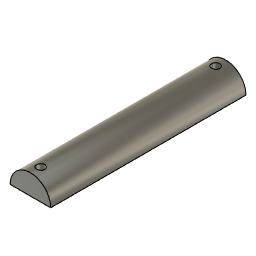
Shaker Fixture v1 (Autodesk Fusion 360 design; units mm, degrees)
Autodesk Fusion 360 part; units mm, degrees
sketch "Sketch1" plane through (0, 0, 0) normal (0, 1, 0) x (1, 0, 0)
  line L0 (0, 0) -> (10, 0)
  line L1 (0, 0) -> (-10, 0)
  arc A0 (-10, 0) -> (10, 0) centre (0, 0) ccw
  dimension "d1" = 10
  dimension "d2" = 10
  constraint coincident L0.start L1.start
  constraint horizontal L0
  constraint parallel L0 L1
  measures "d1" distance of L0.start L0.end
  measures "d2" distance of L0.start L1.end L1.start
extrude "Extrude1" add sketch "Sketch1" along normal blind 96.2
sketch "Sketch2" plane through (0, 0, 0) normal (0, 0, -1) x (1, 0, 0)
  line L0 (10, 0) -> (-10, 0)
  line L1 (-10, 0) -> (-10, -96.2)
  line L2 (-10, -96.2) -> (10, -96.2)
  line L3 (10, -96.2) -> (10, 0)
  line L4 (10, -48.1) -> (-10, -48.1)
  line L5 (10, -48.1) -> (10, -10)
  line L6 (10, -48.1) -> (10, -86.2)
  line L7 (10, -10) -> (10, -5)
  line L8 (10, -5) -> (0, -5)
  circle A0 centre (0, -5) radius 2
  line L9 (10, -86.2) -> (10, -91.2)
  line L10 (10, -91.2) -> (0, -91.2)
  circle A1 centre (0, -91.2) radius 2
  dimension "d6" = 38.1
  dimension "d7" = 38.1
  dimension "d8" = 5
  dimension "d9" = 4
  dimension "d10" = 5
  dimension "d11" = 4
  constraint midpoint L3 L4.start
  constraint midpoint L1 L4.end
  constraint perpendicular L4 L5
  constraint perpendicular L4 L6
  constraint parallel L3 L7
  constraint perpendicular L7 L8
  constraint coincident L8.end A0.centre
  constraint perpendicular L2 L9
  constraint perpendicular L9 L10
  constraint coincident L10.end A1.centre
  measures "d6" distance of L4.start L5.end
  measures "d7" distance of L4.start L6.end
  measures "d8" distance of L5.end L7.end
  measures "d9" diameter of A0
  measures "d10" distance of L6.end L9.end
  measures "d11" diameter of A1
extrude "Extrude2" cut sketch "Sketch2" against normal blind 20.439 contours A0 | A1
